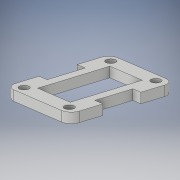
# Autodesk Inventor part: 板子7
Saved by Autodesk Inventor 2017 (Build 210142000, 142)
## iProperties
Part Number: 板子7
Material: 一般
Document SubType Name: Modeling
Designer: User
Density: 1 g/cm^3
Appearance: 預設
Author: User
Autodesk Inventor part; units mm, degrees
ref_plane "YZ Plane" through (0, 0, 0) normal (1, 0, 0) x (0, 1, 0)
ref_plane "XZ Plane" through (0, 0, 0) normal (0, 1, 0) x (-1, 0, 0)
ref_plane "XY Plane" through (0, 0, 0) normal (0, 0, 1) x (1, 0, 0)
sketch "草圖1" plane through (0, 0, 0) normal (0, 1, 0) x (-1, 0, 0)
  line L0 (12, 16.5) -> (-12, 16.5)
  line L1 (-12, -16.5) -> (12, -16.5)
  line L2 (12, -16.5) -> (12, 16.5)
  line L3 (6.1, 11.4) -> (-6.1, 11.4)
  line L4 (-6.1, 11.4) -> (-6.1, -11.4)
  line L5 (-6.1, -11.4) -> (6.1, -11.4)
  line L6 (6.1, -11.4) -> (6.1, 11.4)
  circle A0 centre (8.5, 13.7) radius 1.5
  line L7 (12, 6) -> (9, 6)
  line L8 (9, 6) -> (9, -6)
  line L9 (9, -6) -> (12, -6)
  line L10 (12, -6) -> (12, 6)
  line L11 (0, -23.1) -> (0, 23.1) projected
  line L12 (16.8, 0) -> (-16.8, 0) projected
  circle A1 centre (8.5, -13.7) radius 1.5
  circle A2 centre (-8.5, 13.7) radius 1.5
  line L13 (-12, 6) -> (-9, 6)
  line L14 (-9, 6) -> (-9, -6)
  line L15 (-9, -6) -> (-12, -6)
  circle A3 centre (-8.5, -13.7) radius 1.5
  line L16 (-12, 16.5) -> (-12, 6)
  line L17 (-12, -6) -> (-12, -16.5)
  point P0 (0, 0)
  dimension "d0" = 16.5
  dimension "d1" = 33
  dimension "d2" = 24
  dimension "d4" = 12.2
  dimension "d5" = 22.8
  dimension "d6" = 6.1
  dimension "d7" = 11.4
  dimension "d8" = 3
  dimension "d9" = 3.5
  dimension "d10" = 2.8
  dimension "d11" = 12
  dimension "d12" = 3
  dimension "d13" = 6
  constraints: 32 end point, 7 parallel, 7 symmetric about line, 4 centre point, 4 perpendicular, 3 horizontal, 1 point on line, 3 other
  measures "d0" distance from line of point (0, 0) L1
  measures "d1" distance of L1.end L0.start
  measures "d2" distance of L0.start L0.end
  measures "d4" distance of L3.start L3.end
  measures "d5" distance of L5.end L3.start
  measures "d6" distance from line of point (0, 0) L6
  measures "d7" distance from line of point (0, 0) L3
  measures "d8" diameter of A0
  measures "d9" distance from line of L2 A0.centre
  measures "d10" distance from line of L0 A0.centre
  measures "d11" distance of L7.end L8.end
  measures "d12" distance of L8.end L9.end
  measures "d13" distance from line of point (0, 0) L7
extrude "擠出1" add sketch "草圖1" along normal mid plane 3 contours L2 L7 L8 L12 L6 L3 L11 L0 | L11 L3 L4 L12 L14 L13 L16 L0 | L2 L1 L11 L5 L6 L12 L8 L9 | L4 L5 L11 L1 L17 L15 L14 L12
fillet "圓角1" radius 3 4 edges at (12, 0, 16.5) (-12, 0, 16.5) (-12, 0, -16.5) (12, 0, -16.5)
